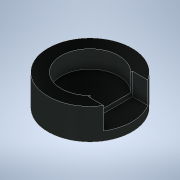
# Autodesk Inventor part: prindere senzor
Saved by Autodesk Inventor 2022 (Build 260153000, 153)
## iProperties
Created: 2022-02-27
Part Number: prindere senzor
Material: Generic
Document SubType Name: Modeling
Designer: Oana
Density: 1 g/cm^3
Appearance: Gunmetal - Polished
Author: Oana
Autodesk Inventor part; units mm, degrees
ref_plane "YZ Plane" through (0, 0, 0) normal (1, 0, 0) x (0, 1, 0)
ref_plane "XZ Plane" through (0, 0, 0) normal (0, 1, 0) x (-1, 0, 0)
ref_plane "XY Plane" through (0, 0, 0) normal (0, 0, 1) x (1, 0, 0)
sketch "Sketch1" plane through (0, 0, 0) normal (0, 1, 0) x (-1, 0, 0)
  circle A0 centre (0, 0) radius 9.5
  line L0 (-3.8533, 8.6834) -> (-3.8533, 38.6834)
  line L1 (-7.8533, -5.3457) -> (-7.8533, 38.6834)
  line L2 (-7.8533, 38.6834) -> (-3.8533, 38.6834)
  line L3 (-5.8533, 7.4826) -> (-5.8533, 50.3065) construction
  line L4 (-3.8533, 38.6834) -> (-7.8533, -5.3457) construction
  line L5 (-7.8533, 38.6834) -> (-3.8533, 8.6834) construction
  line L6 (-2.7738, -9.086) -> (-2.7738, -39.086)
  line L7 (-2.7738, -39.086) -> (-6.7738, -39.086)
  line L8 (-6.7738, -39.086) -> (-6.7738, 6.6608)
  point P0 (-5.8533, 16.6689)
  dimension "d0" = 19
  dimension "d10" = 30
  dimension "d16" = 4
  constraints: 18 end point, 5 point on circle, 3 perpendicular, 3 vertical, 2 parallel, 1 centre point, 1 coincident, 1 horizontal, 1 midpoint, 1 point on line
  measures "d0" diameter of A0
  measures "d10" distance of L0.start L0.end
  measures "d16" distance of L1.end L0.end
extrude "Extrusion1" add sketch "Sketch1" along normal blind 3 contours A0 L8 | L8 A0 L1 | L1 A0
sketch "Sketch2" plane through (0, 3, 0) normal (0, 1, 0) x (1, 0, 0)
  circle A0 centre (0, 0) radius 6.5
  circle A1 centre (0, 0) radius 9.5 projected
  dimension "d3" = 3
  constraints: 1 centre point, 1 coincident
  measures "d3" radial gap between concentric circles of A1 A0
extrude "Extrusion2" add sketch "Sketch2" along normal blind 4
sketch "Sketch3" plane through (0, 7, 0) normal (0, 1, 0) x (1, 0, 0)
  line L0 (4.6242, -5) -> (32.9242, -5)
  line L1 (32.9242, -5) -> (32.9242, 5)
  line L2 (32.9242, 5) -> (4.6242, 5)
  line L3 (4.6242, 5) -> (4.6242, -5)
  line L4 (4.6242, -5) -> (32.9242, 5)
  line L5 (4.6242, 5) -> (32.9242, -5)
  line L6 (0, 0) -> (18.7742, 0)
  dimension "d6" = 10
  dimension "d7" = 28.3
  constraints: 14 end point, 2 horizontal, 2 parallel, 1 coincident, 1 midpoint, 1 perpendicular
  measures "d6" distance of L2.end L0.start
  measures "d7" distance of L1.end L2.end
extrude "Extrusion3" cut sketch "Sketch3" against normal blind 5
body "Solid1"
